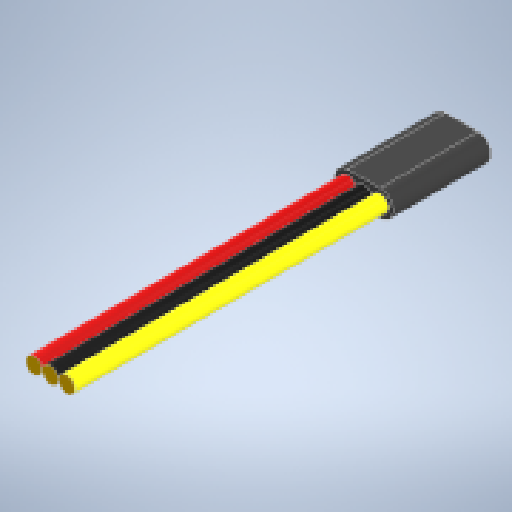
# Autodesk Inventor part: Cables
Saved by Autodesk Inventor 2023.2 (Build 272271000, 271)
## iProperties
Created: 2023-03-04
Part Number: Cables
Material: Rubber
Document SubType Name: Modeling
Designer: Nathan Cai
Density: 0.93 g/cm^3
Appearance: Rubber - Black
Author: Nathan Cai
Autodesk Inventor part; units mm, degrees
ref_plane "YZ Plane" through (0, 0, 0) normal (1, 0, 0) x (0, 1, 0)
ref_plane "XZ Plane" through (0, 0, 0) normal (0, 1, 0) x (-1, 0, 0)
ref_plane "XY Plane" through (0, 0, 0) normal (0, 0, 1) x (1, 0, 0)
sketch "Sketch1" plane through (0, 0, 0) normal (0, 0, 1) x (1, 0, 0)
  line L0 (-2.5, 0) -> (2.5, 0) construction
  line L1 (-2.5, -2) -> (2.5, -2)
  line L2 (2.5, 2) -> (-2.5, 2)
  arc A0 (-2.5, 2) -> (-2.5, -2) centre (-2.5, 0) ccw
  arc A1 (2.5, -2) -> (2.5, 2) centre (2.5, 0) ccw
  point P0 (0, 0)
  dimension "d0" = 2.5
  dimension "d1" = 4
  constraints: 8 end point, 4 point on circle, 4 tangent, 2 centre point, 1 horizontal, 1 midpoint, 1 parallel
  measures "d0" distance of point (0, 0) L0.end
  measures "d1" diameter of A1
extrude "Extrusion1" add sketch "Sketch1" along normal blind 15
sketch "Sketch2" plane through (0, 0, 15) normal (0, 0, 1) x (1, 0, 0)
  circle A0 centre (0, 0) radius 1.25
  line L0 (0, 0) -> (4.5, 0) construction
  arc A1 (2.5, -2) -> (2.5, 2) centre (2.5, 0) ccw projected
  circle A2 centre (2.5, 0) radius 1.25
  circle A3 centre (-2.5, 0) radius 1.25
  point P0 (-1.25, 0)
  point P1 (1.25, 0)
  dimension "d4" = 2.5
  dimension "d5" = 2.5
  dimension "d8" = 360
  constraints: 3 centre point, 2 coincident, 2 end point, 1 horizontal, 1 point on circle, 5 other
  measures "d4" diameter of A0
  measures "d5" diameter of A2
extrude "Extrusion2" add sketch "Sketch2" along normal blind 48
body "Solid1"
